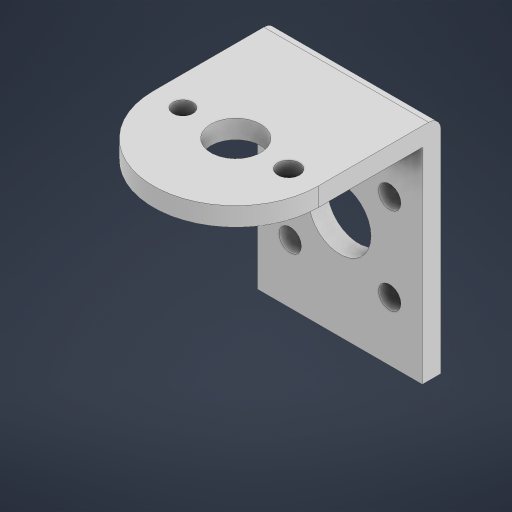
# Autodesk Inventor part: bracket jga
Saved by Autodesk Inventor 2024.3 (Build 283343000, 343)
## iProperties
Created: 2025-06-12
Part Number: bracket jga
Material: Generic
Document SubType Name: Modeling
Designer: Akbar Syihabuddin
Density: 1 g/cm^3
Appearance: Default
Author: Akbar Syihabuddin
Autodesk Inventor part; units mm, degrees
ref_plane "YZ Plane" through (0, 0, 0) normal (1, 0, 0) x (0, 1, 0)
ref_plane "XZ Plane" through (0, 0, 0) normal (0, 1, 0) x (-1, 0, 0)
ref_plane "XY Plane" through (0, 0, 0) normal (0, 0, 1) x (1, 0, 0)
sketch "Sketch1" plane through (0, 0, 0) normal (0, 1, 0) x (-1, 0, 0)
  line L0 (0, 0) -> (26.5, 0)
  line L1 (26.5, 0) -> (26.5, -33)
  line L2 (26.5, -33) -> (0, -33)
  line L3 (0, -33) -> (0, 0)
  line L4 (26.5, -33) -> (26.5, -30)
  line L5 (26.5, -30) -> (0, -30)
  circle A0 centre (13.25, -13.25) radius 4
  arc A1 (22.5449, -12.2666) -> (20.6583, -12.6119) centre (21.75, -13.25) ccw
  circle A2 centre (21.75, -13.25) radius 1.6
  circle A3 centre (4.75, -13.25) radius 1.75
  circle A4 centre (4.75, -13.25) radius 1.6
  circle A5 centre (13.25, -13.25) radius 13.25
  line L6 (13.25, -13.25) -> (13.25, 0)
  line L7 (13.25, 0) -> (13.25, -13.25)
  point P0 (0, -13.25)
  point P1 (26.5, -13.25)
  dimension "d9" = 26.5
  dimension "d3" = 26.5
  dimension "d4" = 33
  dimension "d5" = 3
  dimension "d6" = 8
  dimension "d7" = 3.2
  dimension "d8" = 3.2
  dimension "d10" = 13.25
  constraints: 16 end point, 5 centre point, 4 coincident, 2 parallel, 2 perpendicular, 2 point on circle, 2 point on line, 2 vertical, 1 horizontal, 1 midpoint, 3 other
  measures "d3" distance of L1.end L2.end
  measures "d4" distance of L0.end L1.end
  measures "d5" distance of L1.end L4.end
  measures "d6" diameter of A0
  measures "d7" diameter of A2
  measures "d8" diameter of A4
  measures "d10" distance of L7.start L7.end
extrude "Extrusion1" add sketch "Sketch1" along normal blind 3 contours A5 | A5 L1 L5 L3 | L5 L1 L2 L3
sketch "Sketch2" plane through (0, 0, 0) normal (0, -1, 0) x (1, 0, 0)
  line L0 (0, -33) -> (-26.5, -33) projected
  line L1 (0, -13.25) -> (0, -33) projected
  line L2 (-26.5, -33) -> (0, -33)
  line L3 (0, -33) -> (0, -30)
  line L4 (0, -30) -> (-26.5, -30)
  line L5 (-26.5, -30) -> (-26.5, -33)
  point P0 (0, 0)
  dimension "d13" = 3
  constraints: 8 end point, 2 parallel, 1 horizontal, 1 perpendicular, 1 point on line
  measures "d13" distance of L3.end L2.end
extrude "Extrusion2" add sketch "Sketch2" along normal blind 33
fillet "Fillet1" radius 2 1 edges at (-13.25, 3, -33)
sketch "Sketch3" plane through (-26.5, 0, -30) normal (0, 0, 1) x (1, 0, 0)
  line L0 (26.5, -33) -> (0, -33) projected
  line L1 (13.25, -33) -> (13.25, 0)
  line L2 (0, 0) -> (0, -33) projected
  line L3 (0, -16.5) -> (26.5, -16.5)
  line L4 (26.5, 0) -> (26.5, -33) projected
  circle A0 centre (13.25, -16.5) radius 5
  line L5 (0, -16.5) -> (0, -23.5)
  line L6 (13.25, -33) -> (5.25, -33)
  circle A1 centre (5.25, -23.5) radius 1.8
  circle A2 centre (5.25, -9.5) radius 1.8
  circle A3 centre (21.25, -23.5) radius 1.8
  circle A4 centre (21.25, -9.5) radius 1.8
  dimension "d17" = 10
  dimension "d18" = 7
  dimension "d19" = 8
  dimension "d20" = 3.6
  dimension "d23" = 14
  dimension "d26" = 16
  constraints: 8 end point, 5 centre point, 4 midpoint, 2 point on line, 2 vertical, 1 horizontal, 6 other
  measures "d17" diameter of A0
  measures "d18" distance of L3.start L5.end
  measures "d19" distance of L1.start L6.end
  measures "d20" diameter of A1
  measures "d23" distance of A1.centre A2.centre
  measures "d26" distance of A1.centre A3.centre
extrude "Extrusion3" cut sketch "Sketch3" against normal blind 33 contours A0 L3 L1 | L1 L3 A0 | L3 L1 A0 | L3 A0 L1 | A1 | A2 | A3 | A4
body "Solid1"
